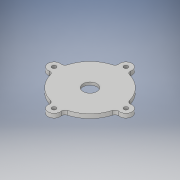
# Autodesk Inventor part: topPlateGB
Saved by Autodesk Inventor 2019 (Build 230136000, 136)
## iProperties
Created: 2019-10-26
Part Number: topPlateGB
Material: Generic
Document SubType Name: Modeling
Designer: test
Density: 1 g/cm^3
Appearance: Default
Author: test
Autodesk Inventor part; units mm, degrees
ref_plane "YZ Plane" through (0, 0, 0) normal (1, 0, 0) x (0, 1, 0)
ref_plane "XZ Plane" through (0, 0, 0) normal (0, 1, 0) x (-1, 0, 0)
ref_plane "XY Plane" through (0, 0, 0) normal (0, 0, 1) x (1, 0, 0)
sketch "Sketch1" plane through (0, 0, 0) normal (0, 1, 0) x (-1, 0, 0)
  circle A0 centre (33.02, 0) radius 1.778
  circle A1 centre (-33.02, 0) radius 1.778
  circle A2 centre (0, 33.02) radius 1.778
  circle A3 centre (0, -33.02) radius 1.778
  arc A4 (23.784909, -5.42928) -> (23.805274, -5.339279) centre (0, 0) ccw
  arc A5 (23.784909, -5.42928) -> (23.931742, -5.761352) centre (24.080982, -5.496864) ccw
  arc A6 (25.319623, -6.710384) -> (23.931742, -5.761352) centre (19.12448, -14.280927) ccw
  arc A7 (25.143294, -7.34352) -> (25.319623, -6.710384) centre (0, 0) ccw
  arc A8 (23.464649, -7.438525) -> (25.143294, -7.34352) centre (23.753261, 2.339492) ccw
  arc A9 (23.464649, -7.438525) -> (23.167304, -7.646894) centre (23.45569, -7.742082) ccw
  arc A10 (23.138215, -7.734466) -> (23.167304, -7.646894) centre (0, 0) ccw
  arc A11 (23.138215, -7.734466) -> (23.251792, -8.079331) centre (23.426239, -7.830744) ccw
  arc A12 (24.539969, -9.159828) -> (23.251792, -8.079331) centre (17.632615, -16.086687) ccw
  arc A13 (24.302432, -9.772633) -> (24.539969, -9.159828) centre (0, 0) ccw
  arc A14 (22.622558, -9.702644) -> (24.302432, -9.772633) centre (23.868193, 0) ccw
  arc A15 (22.622558, -9.702644) -> (22.306221, -9.880865) centre (22.583887, -10.003861) ccw
  arc A16 (22.268688, -9.965164) -> (22.306221, -9.880865) centre (0, 0) ccw
  arc A17 (22.268688, -9.965164) -> (22.347916, -10.319501) centre (22.545888, -10.08921) ccw
  arc A18 (23.523982, -11.521059) -> (22.347916, -10.319501) centre (15.970938, -17.737524) ccw
  arc A19 (23.227523, -12.10763) -> (23.523982, -11.521059) centre (0, 0) ccw
  arc A20 (21.562599, -11.873322) -> (23.227523, -12.10763) centre (23.753261, -2.339492) ccw
  arc A21 (21.562599, -11.873322) -> (21.230316, -12.019678) centre (21.49459, -12.169298) ccw
  arc A22 (21.184702, -12.099892) -> (21.230316, -12.019678) centre (0, 0) ccw
  arc A23 (21.184702, -12.099892) -> (21.228816, -12.460288) centre (21.448408, -12.250511) ccw
  arc A24 (22.281447, -13.771335) -> (21.228816, -12.460288) centre (14.155452, -19.217539) ccw
  arc A25 (21.928921, -14.326024) -> (22.281447, -13.771335) centre (0, 0) ccw
  arc A26 (20.29498, -13.929653) -> (21.928921, -14.326024) centre (23.409572, -4.656453) ccw
  arc A27 (20.29498, -13.929653) -> (19.949952, -14.042734) centre (20.198288, -14.217538) ccw
  arc A28 (19.896695, -14.118092) -> (19.949952, -14.042734) centre (0, 0) ccw
  arc A29 (19.896695, -14.118092) -> (19.905272, -14.481076) centre (20.144368, -14.293833) ccw
  arc A30 (20.824328, -15.888986) -> (19.905272, -14.481076) centre (12.203642, -20.512478) ccw
  arc A31 (20.419132, -16.40645) -> (20.824328, -15.888986) centre (0, 0) ccw
  arc A32 (18.831909, -15.851834) -> (20.419132, -16.40645) centre (22.840436, -6.928571) ccw
  arc A33 (18.831909, -15.851834) -> (18.477459, -15.930552) centre (18.707465, -16.128855) ccw
  arc A34 (18.417072, -16.000326) -> (18.477459, -15.930552) centre (0, 0) ccw
  arc A35 (18.417072, -16.000326) -> (18.390029, -16.362404) centre (18.646326, -16.199497) ccw
  arc A36 (19.166661, -17.853618) -> (18.390029, -16.362404) centre (10.134303, -21.609871) ccw
  arc A37 (18.712695, -18.328873) -> (19.166661, -17.853618) centre (0, 0) ccw
  arc A38 (17.187477, -17.621353) -> (18.712695, -18.328873) centre (22.051335, -9.133962) ccw
  arc A39 (17.187477, -17.621353) -> (16.827018, -17.66495) centre (17.036479, -17.884842) ccw
  arc A40 (16.760082, -17.728469) -> (16.827018, -17.66495) centre (0, 0) ccw
  arc A41 (16.760082, -17.728469) -> (16.69768, -18.086153) centre (16.968711, -17.949152) ccw
  arc A42 (17.324407, -19.646309) -> (16.69768, -18.086153) centre (7.967366, -22.499149) ccw
  arc A43 (16.826044, -20.07478) -> (17.324407, -19.646309) centre (0, 0) ccw
  arc A44 (15.37752, -19.221168) -> (16.826044, -20.07478) centre (21.049867, -11.251388) ccw
  arc A45 (15.37752, -19.221168) -> (15.014523, -19.229224) centre (15.201423, -19.468589) ccw
  arc A46 (14.941684, -19.285877) -> (15.014523, -19.229224) centre (0, 0) ccw
  arc A47 (14.941684, -19.285877) -> (14.844523, -19.635722) centre (15.127677, -19.525946) ccw
  arc A48 (15.315311, -21.249795) -> (14.844523, -19.635722) centre (5.723699, -23.171748) ccw
  arc A49 (14.77735, -21.627355) -> (15.315311, -21.249795) centre (0, 0) ccw
  arc A50 (13.419469, -20.635874) -> (14.77735, -21.627355) centre (19.845677, -13.260457) ccw
  arc A51 (13.419469, -20.635874) -> (13.05743, -20.608311) centre (13.219969, -20.864842) ccw
  arc A52 (12.979389, -20.657551) -> (13.05743, -20.608311) centre (0, 0) ccw
  arc A53 (12.979389, -20.657551) -> (12.848405, -20.996188) centre (13.140956, -20.914695) ccw
  arc A54 (13.158719, -22.648635) -> (12.848405, -20.996188) centre (3.424909, -23.62119) ccw
  arc A55 (12.586341, -22.971647) -> (13.158719, -22.648635) centre (0, 0) ccw
  arc A56 (11.332181, -21.851844) -> (12.586341, -22.971647) centre (18.450362, -15.141821) ccw
  arc A57 (11.332181, -21.851844) -> (10.974588, -21.788928) centre (11.111199, -22.060156) ccw
  arc A58 (10.892096, -21.830282) -> (10.974588, -21.788928) centre (0, 0) ccw
  arc A59 (10.892096, -21.830282) -> (10.728551, -22.15445) centre (11.02768, -22.102024) ccw
  arc A60 (10.875402, -23.829355) -> (10.728551, -22.15445) centre (1.093136, -23.843147) ccw
  arc A61 (10.274119, -24.094709) -> (10.875402, -23.829355) centre (0, 0) ccw
  arc A62 (9.135758, -22.85737) -> (10.274119, -24.094709) centre (16.877361, -16.877361) ccw
  arc A63 (9.135758, -22.85737) -> (8.786054, -22.759706) centre (8.895422, -23.043018) ccw
  arc A64 (8.699906, -22.792775) -> (8.786054, -22.759706) centre (0, 0) ccw
  arc A65 (8.699906, -22.792775) -> (8.505374, -23.099352) centre (8.808202, -23.076499) ccw
  arc A66 (8.487348, -24.780586) -> (8.505374, -23.099352) centre (-1.249165, -23.835482) ccw
  arc A67 (7.862952, -24.985726) -> (8.487348, -24.780586) centre (0, 0) ccw
  arc A68 (6.851353, -23.642766) -> (7.862952, -24.985726) centre (15.141821, -18.450362) ccw
  arc A69 (6.851353, -23.642766) -> (6.512905, -23.511296) centre (6.593977, -23.803963) ccw
  arc A70 (6.42393, -23.535762) -> (6.512905, -23.511296) centre (0, 0) ccw
  arc A71 (6.42393, -23.535762) -> (6.200286, -23.821794) centre (6.503895, -23.828734) ccw
  arc A72 (6.017557, -25.493167) -> (6.200286, -23.821794) centre (-3.579436, -23.598268) ccw
  arc A73 (5.37606, -25.636117) -> (6.017557, -25.493167) centre (0, 0) ccw
  arc A74 (4.500966, -24.20047) -> (5.37606, -25.636117) centre (13.260457, -19.845677) ccw
  arc A75 (4.500966, -24.20047) -> (4.177034, -24.036459) centre (4.229029, -24.335663) ccw
  arc A76 (4.086089, -24.052086) -> (4.177034, -24.036459) centre (0, 0) ccw
  arc A77 (4.086089, -24.052086) -> (3.835486, -24.31482) centre (4.136953, -24.351485) ccw
  arc A78 (3.489814, -25.960234) -> (3.835486, -24.31482) centre (-5.875234, -23.13379) ccw
  arc A79 (2.837394, -26.039619) -> (3.489814, -25.960234) centre (0, 0) ccw
  arc A80 (2.107231, -24.52511) -> (2.837394, -26.039619) centre (11.251388, -21.049867) ccw
  arc A81 (2.107231, -24.52511) -> (1.800935, -24.330138) centre (1.823353, -24.632998) ccw
  arc A82 (1.708897, -24.336775) -> (1.800935, -24.330138) centre (0, 0) ccw
  arc A83 (1.708897, -24.336775) -> (1.433747, -24.573681) centre (1.730169, -24.639718) ccw
  arc A84 (0.928462, -26.17729) -> (1.433747, -24.573681) centre (-8.114452, -22.446521) ccw
  arc A85 (0.271403, -26.192344) -> (0.928462, -26.17729) centre (0, 0) ccw
  arc A86 (-0.306797, -24.613559) -> (0.271403, -26.192344) centre (9.133962, -22.051335) ccw
  arc A87 (-0.306797, -24.613559) -> (-0.592507, -24.389504) centre (-0.599883, -24.693103) ccw
  arc A88 (-0.684753, -24.387088) -> (-0.592507, -24.389504) centre (0, 0) ccw
  arc A89 (-0.684753, -24.387088) -> (-0.981798, -24.595884) centre (-0.693277, -24.690658) ccw
  arc A90 (-1.641832, -26.142244) -> (-0.981798, -24.595884) centre (-10.275522, -21.543079) ccw
  arc A91 (-2.297203, -26.092823) -> (-1.641832, -26.142244) centre (0, 0) ccw
  arc A92 (-2.71787, -24.464967) -> (-2.297203, -26.092823) centre (6.928571, -22.840436) ccw
  arc A93 (-2.71787, -24.464967) -> (-2.980244, -24.213986) centre (-3.017342, -24.5154) ccw
  arc A94 (-3.071808, -24.20254) -> (-2.980244, -24.213986) centre (0, 0) ccw
  arc A95 (-3.071808, -24.20254) -> (-3.387889, -24.381215) centre (-3.110046, -24.503812) ccw
  arc A96 (-4.196314, -25.855434) -> (-3.387889, -24.381215) centre (-12.337634, -20.432166) ccw
  arc A97 (-4.843685, -25.742013) -> (-4.196314, -25.855434) centre (0, 0) ccw
  arc A98 (-5.102769, -24.080764) -> (-4.843685, -25.742013) centre (4.656453, -23.409572) ccw
  arc A99 (-5.102769, -24.080764) -> (-5.339279, -23.805274) centre (-5.405742, -24.101601) ccw
  arc A100 (-5.42928, -23.784909) -> (-5.339279, -23.805274) centre (0, 0) ccw
  arc A101 (-5.42928, -23.784909) -> (-5.761352, -23.931742) centre (-5.496864, -24.080982) ccw
  arc A102 (-6.710384, -25.319623) -> (-5.761352, -23.931742) centre (-14.280927, -19.12448) ccw
  arc A103 (-7.34352, -25.143294) -> (-6.710384, -25.319623) centre (0, 0) ccw
  arc A104 (-7.438525, -23.464649) -> (-7.34352, -25.143294) centre (2.339492, -23.753261) ccw
  arc A105 (-7.438525, -23.464649) -> (-7.646894, -23.167304) centre (-7.742082, -23.45569) ccw
  arc A106 (-7.734466, -23.138215) -> (-7.646894, -23.167304) centre (0, 0) ccw
  arc A107 (-7.734466, -23.138215) -> (-8.079331, -23.251792) centre (-7.830744, -23.426239) ccw
  arc A108 (-9.159828, -24.539969) -> (-8.079331, -23.251792) centre (-16.086687, -17.632615) ccw
  arc A109 (-9.772633, -24.302432) -> (-9.159828, -24.539969) centre (0, 0) ccw
  arc A110 (-9.702644, -22.622558) -> (-9.772633, -24.302432) centre (0, -23.868193) ccw
  arc A111 (-9.702644, -22.622558) -> (-9.880865, -22.306221) centre (-10.003861, -22.583887) ccw
  arc A112 (-9.965164, -22.268688) -> (-9.880865, -22.306221) centre (0, 0) ccw
  arc A113 (-9.965164, -22.268688) -> (-10.319501, -22.347916) centre (-10.08921, -22.545888) ccw
  arc A114 (-11.521059, -23.523982) -> (-10.319501, -22.347916) centre (-17.737524, -15.970938) ccw
  arc A115 (-12.10763, -23.227523) -> (-11.521059, -23.523982) centre (0, 0) ccw
  arc A116 (-11.873322, -21.562599) -> (-12.10763, -23.227523) centre (-2.339492, -23.753261) ccw
  arc A117 (-11.873322, -21.562599) -> (-12.019678, -21.230316) centre (-12.169298, -21.49459) ccw
  arc A118 (-12.099892, -21.184702) -> (-12.019678, -21.230316) centre (0, 0) ccw
  arc A119 (-12.099892, -21.184702) -> (-12.460288, -21.228816) centre (-12.250511, -21.448408) ccw
  arc A120 (-13.771335, -22.281447) -> (-12.460288, -21.228816) centre (-19.217539, -14.155452) ccw
  arc A121 (-14.326024, -21.928921) -> (-13.771335, -22.281447) centre (0, 0) ccw
  arc A122 (-13.929653, -20.29498) -> (-14.326024, -21.928921) centre (-4.656453, -23.409572) ccw
  arc A123 (-13.929653, -20.29498) -> (-14.042734, -19.949952) centre (-14.217538, -20.198288) ccw
  arc A124 (-14.118092, -19.896695) -> (-14.042734, -19.949952) centre (0, 0) ccw
  arc A125 (-14.118092, -19.896695) -> (-14.481076, -19.905272) centre (-14.293833, -20.144368) ccw
  arc A126 (-15.888986, -20.824328) -> (-14.481076, -19.905272) centre (-20.512478, -12.203642) ccw
  arc A127 (-16.40645, -20.419132) -> (-15.888986, -20.824328) centre (0, 0) ccw
  arc A128 (-15.851834, -18.831909) -> (-16.40645, -20.419132) centre (-6.928571, -22.840436) ccw
  arc A129 (-15.851834, -18.831909) -> (-15.930552, -18.477459) centre (-16.128855, -18.707465) ccw
  arc A130 (-16.000326, -18.417072) -> (-15.930552, -18.477459) centre (0, 0) ccw
  arc A131 (-16.000326, -18.417072) -> (-16.362404, -18.390029) centre (-16.199497, -18.646326) ccw
  arc A132 (-17.853618, -19.166661) -> (-16.362404, -18.390029) centre (-21.609871, -10.134303) ccw
  arc A133 (-18.328873, -18.712695) -> (-17.853618, -19.166661) centre (0, 0) ccw
  arc A134 (-17.621353, -17.187477) -> (-18.328873, -18.712695) centre (-9.133962, -22.051335) ccw
  arc A135 (-17.621353, -17.187477) -> (-17.66495, -16.827018) centre (-17.884842, -17.036479) ccw
  arc A136 (-17.728469, -16.760082) -> (-17.66495, -16.827018) centre (0, 0) ccw
  arc A137 (-17.728469, -16.760082) -> (-18.086153, -16.69768) centre (-17.949152, -16.968711) ccw
  arc A138 (-19.646309, -17.324407) -> (-18.086153, -16.69768) centre (-22.499149, -7.967366) ccw
  arc A139 (-20.07478, -16.826044) -> (-19.646309, -17.324407) centre (0, 0) ccw
  arc A140 (-19.221168, -15.37752) -> (-20.07478, -16.826044) centre (-11.251388, -21.049867) ccw
  arc A141 (-19.221168, -15.37752) -> (-19.229224, -15.014523) centre (-19.468589, -15.201423) ccw
  arc A142 (-19.285877, -14.941684) -> (-19.229224, -15.014523) centre (0, 0) ccw
  arc A143 (-19.285877, -14.941684) -> (-19.635722, -14.844523) centre (-19.525946, -15.127677) ccw
  arc A144 (-21.249795, -15.315311) -> (-19.635722, -14.844523) centre (-23.171748, -5.723699) ccw
  arc A145 (-21.627355, -14.77735) -> (-21.249795, -15.315311) centre (0, 0) ccw
  arc A146 (-20.635874, -13.419469) -> (-21.627355, -14.77735) centre (-13.260457, -19.845677) ccw
  arc A147 (-20.635874, -13.419469) -> (-20.608311, -13.05743) centre (-20.864842, -13.219969) ccw
  arc A148 (-20.657551, -12.979389) -> (-20.608311, -13.05743) centre (0, 0) ccw
  arc A149 (-20.657551, -12.979389) -> (-20.996188, -12.848405) centre (-20.914695, -13.140956) ccw
  arc A150 (-22.648635, -13.158719) -> (-20.996188, -12.848405) centre (-23.62119, -3.424909) ccw
  arc A151 (-22.971647, -12.586341) -> (-22.648635, -13.158719) centre (0, 0) ccw
  arc A152 (-21.851844, -11.332181) -> (-22.971647, -12.586341) centre (-15.141821, -18.450362) ccw
  arc A153 (-21.851844, -11.332181) -> (-21.788928, -10.974588) centre (-22.060156, -11.111199) ccw
  arc A154 (-21.830282, -10.892096) -> (-21.788928, -10.974588) centre (0, 0) ccw
  arc A155 (-21.830282, -10.892096) -> (-22.15445, -10.728551) centre (-22.102024, -11.02768) ccw
  arc A156 (-23.829355, -10.875402) -> (-22.15445, -10.728551) centre (-23.843147, -1.093136) ccw
  arc A157 (-24.094709, -10.274119) -> (-23.829355, -10.875402) centre (0, 0) ccw
  arc A158 (-22.85737, -9.135758) -> (-24.094709, -10.274119) centre (-16.877361, -16.877361) ccw
  arc A159 (-22.85737, -9.135758) -> (-22.759706, -8.786054) centre (-23.043018, -8.895422) ccw
  arc A160 (-22.792775, -8.699906) -> (-22.759706, -8.786054) centre (0, 0) ccw
  arc A161 (-22.792775, -8.699906) -> (-23.099352, -8.505374) centre (-23.076499, -8.808202) ccw
  arc A162 (-24.780586, -8.487348) -> (-23.099352, -8.505374) centre (-23.835482, 1.249165) ccw
  arc A163 (-24.985726, -7.862952) -> (-24.780586, -8.487348) centre (0, 0) ccw
  arc A164 (-23.642766, -6.851353) -> (-24.985726, -7.862952) centre (-18.450362, -15.141821) ccw
  arc A165 (-23.642766, -6.851353) -> (-23.511296, -6.512905) centre (-23.803963, -6.593977) ccw
  arc A166 (-23.535762, -6.42393) -> (-23.511296, -6.512905) centre (0, 0) ccw
  arc A167 (-23.535762, -6.42393) -> (-23.821794, -6.200286) centre (-23.828734, -6.503895) ccw
  arc A168 (-25.493167, -6.017557) -> (-23.821794, -6.200286) centre (-23.598268, 3.579436) ccw
  arc A169 (-25.636117, -5.37606) -> (-25.493167, -6.017557) centre (0, 0) ccw
  arc A170 (-24.20047, -4.500966) -> (-25.636117, -5.37606) centre (-19.845677, -13.260457) ccw
  arc A171 (-24.20047, -4.500966) -> (-24.036459, -4.177034) centre (-24.335663, -4.229029) ccw
  arc A172 (-24.052086, -4.086089) -> (-24.036459, -4.177034) centre (0, 0) ccw
  arc A173 (-24.052086, -4.086089) -> (-24.31482, -3.835486) centre (-24.351485, -4.136953) ccw
  arc A174 (-25.960234, -3.489814) -> (-24.31482, -3.835486) centre (-23.13379, 5.875234) ccw
  arc A175 (-26.039619, -2.837394) -> (-25.960234, -3.489814) centre (0, 0) ccw
  arc A176 (-24.52511, -2.107231) -> (-26.039619, -2.837394) centre (-21.049867, -11.251388) ccw
  arc A177 (-24.52511, -2.107231) -> (-24.330138, -1.800935) centre (-24.632998, -1.823353) ccw
  arc A178 (-24.336775, -1.708897) -> (-24.330138, -1.800935) centre (0, 0) ccw
  arc A179 (-24.336775, -1.708897) -> (-24.573681, -1.433747) centre (-24.639718, -1.730169) ccw
  arc A180 (-26.17729, -0.928462) -> (-24.573681, -1.433747) centre (-22.446521, 8.114452) ccw
  arc A181 (-26.192344, -0.271403) -> (-26.17729, -0.928462) centre (0, 0) ccw
  arc A182 (-24.613559, 0.306797) -> (-26.192344, -0.271403) centre (-22.051335, -9.133962) ccw
  arc A183 (-24.613559, 0.306797) -> (-24.389504, 0.592507) centre (-24.693103, 0.599883) ccw
  arc A184 (-24.387088, 0.684753) -> (-24.389504, 0.592507) centre (0, 0) ccw
  arc A185 (-24.387088, 0.684753) -> (-24.595884, 0.981798) centre (-24.690658, 0.693277) ccw
  arc A186 (-26.142244, 1.641832) -> (-24.595884, 0.981798) centre (-21.543079, 10.275522) ccw
  arc A187 (-26.092823, 2.297203) -> (-26.142244, 1.641832) centre (0, 0) ccw
  arc A188 (-24.464967, 2.71787) -> (-26.092823, 2.297203) centre (-22.840436, -6.928571) ccw
  arc A189 (-24.464967, 2.71787) -> (-24.213986, 2.980244) centre (-24.5154, 3.017342) ccw
  arc A190 (-24.20254, 3.071808) -> (-24.213986, 2.980244) centre (0, 0) ccw
  arc A191 (-24.20254, 3.071808) -> (-24.381215, 3.387889) centre (-24.503812, 3.110046) ccw
  arc A192 (-25.855434, 4.196314) -> (-24.381215, 3.387889) centre (-20.432166, 12.337634) ccw
  arc A193 (-25.742013, 4.843685) -> (-25.855434, 4.196314) centre (0, 0) ccw
  arc A194 (-24.080764, 5.102769) -> (-25.742013, 4.843685) centre (-23.409572, -4.656453) ccw
  arc A195 (-24.080764, 5.102769) -> (-23.805274, 5.339279) centre (-24.101601, 5.405742) ccw
  arc A196 (-23.784909, 5.42928) -> (-23.805274, 5.339279) centre (0, 0) ccw
  arc A197 (-23.784909, 5.42928) -> (-23.931742, 5.761352) centre (-24.080982, 5.496864) ccw
  arc A198 (-25.319623, 6.710384) -> (-23.931742, 5.761352) centre (-19.12448, 14.280927) ccw
  arc A199 (-25.143294, 7.34352) -> (-25.319623, 6.710384) centre (0, 0) ccw
  arc A200 (-23.464649, 7.438525) -> (-25.143294, 7.34352) centre (-23.753261, -2.339492) ccw
  arc A201 (-23.464649, 7.438525) -> (-23.167304, 7.646894) centre (-23.45569, 7.742082) ccw
  arc A202 (-23.138215, 7.734466) -> (-23.167304, 7.646894) centre (0, 0) ccw
  arc A203 (-23.138215, 7.734466) -> (-23.251792, 8.079331) centre (-23.426239, 7.830744) ccw
  arc A204 (-24.539969, 9.159828) -> (-23.251792, 8.079331) centre (-17.632615, 16.086687) ccw
  arc A205 (-24.302432, 9.772633) -> (-24.539969, 9.159828) centre (0, 0) ccw
  arc A206 (-22.622558, 9.702644) -> (-24.302432, 9.772633) centre (-23.868193, 0) ccw
  arc A207 (-22.622558, 9.702644) -> (-22.306221, 9.880865) centre (-22.583887, 10.003861) ccw
  arc A208 (-22.268688, 9.965164) -> (-22.306221, 9.880865) centre (0, 0) ccw
  arc A209 (-22.268688, 9.965164) -> (-22.347916, 10.319501) centre (-22.545888, 10.08921) ccw
  arc A210 (-23.523982, 11.521059) -> (-22.347916, 10.319501) centre (-15.970938, 17.737524) ccw
  arc A211 (-23.227523, 12.10763) -> (-23.523982, 11.521059) centre (0, 0) ccw
  arc A212 (-21.562599, 11.873322) -> (-23.227523, 12.10763) centre (-23.753261, 2.339492) ccw
  arc A213 (-21.562599, 11.873322) -> (-21.230316, 12.019678) centre (-21.49459, 12.169298) ccw
  arc A214 (-21.184702, 12.099892) -> (-21.230316, 12.019678) centre (0, 0) ccw
  arc A215 (-21.184702, 12.099892) -> (-21.228816, 12.460288) centre (-21.448408, 12.250511) ccw
  arc A216 (-22.281447, 13.771335) -> (-21.228816, 12.460288) centre (-14.155452, 19.217539) ccw
  arc A217 (-21.928921, 14.326024) -> (-22.281447, 13.771335) centre (0, 0) ccw
  arc A218 (-20.29498, 13.929653) -> (-21.928921, 14.326024) centre (-23.409572, 4.656453) ccw
  arc A219 (-20.29498, 13.929653) -> (-19.949952, 14.042734) centre (-20.198288, 14.217538) ccw
  arc A220 (-19.896695, 14.118092) -> (-19.949952, 14.042734) centre (0, 0) ccw
  arc A221 (-19.896695, 14.118092) -> (-19.905272, 14.481076) centre (-20.144368, 14.293833) ccw
  arc A222 (-20.824328, 15.888986) -> (-19.905272, 14.481076) centre (-12.203642, 20.512478) ccw
  arc A223 (-20.419132, 16.40645) -> (-20.824328, 15.888986) centre (0, 0) ccw
  arc A224 (-18.831909, 15.851834) -> (-20.419132, 16.40645) centre (-22.840436, 6.928571) ccw
  arc A225 (-18.831909, 15.851834) -> (-18.477459, 15.930552) centre (-18.707465, 16.128855) ccw
  arc A226 (-18.417072, 16.000326) -> (-18.477459, 15.930552) centre (0, 0) ccw
  arc A227 (-18.417072, 16.000326) -> (-18.390029, 16.362404) centre (-18.646326, 16.199497) ccw
  arc A228 (-19.166661, 17.853618) -> (-18.390029, 16.362404) centre (-10.134303, 21.609871) ccw
  arc A229 (-18.712695, 18.328873) -> (-19.166661, 17.853618) centre (0, 0) ccw
  arc A230 (-17.187477, 17.621353) -> (-18.712695, 18.328873) centre (-22.051335, 9.133962) ccw
  arc A231 (-17.187477, 17.621353) -> (-16.827018, 17.66495) centre (-17.036479, 17.884842) ccw
  arc A232 (-16.760082, 17.728469) -> (-16.827018, 17.66495) centre (0, 0) ccw
  arc A233 (-16.760082, 17.728469) -> (-16.69768, 18.086153) centre (-16.968711, 17.949152) ccw
  arc A234 (-17.324407, 19.646309) -> (-16.69768, 18.086153) centre (-7.967366, 22.499149) ccw
  arc A235 (-16.826044, 20.07478) -> (-17.324407, 19.646309) centre (0, 0) ccw
  arc A236 (-15.37752, 19.221168) -> (-16.826044, 20.07478) centre (-21.049867, 11.251388) ccw
  arc A237 (-15.37752, 19.221168) -> (-15.014523, 19.229224) centre (-15.201423, 19.468589) ccw
  arc A238 (-14.941684, 19.285877) -> (-15.014523, 19.229224) centre (0, 0) ccw
  arc A239 (-14.941684, 19.285877) -> (-14.844523, 19.635722) centre (-15.127677, 19.525946) ccw
  arc A240 (-15.315311, 21.249795) -> (-14.844523, 19.635722) centre (-5.723699, 23.171748) ccw
  arc A241 (-14.77735, 21.627355) -> (-15.315311, 21.249795) centre (0, 0) ccw
  arc A242 (-13.419469, 20.635874) -> (-14.77735, 21.627355) centre (-19.845677, 13.260457) ccw
  arc A243 (-13.419469, 20.635874) -> (-13.05743, 20.608311) centre (-13.219969, 20.864842) ccw
  arc A244 (-12.979389, 20.657551) -> (-13.05743, 20.608311) centre (0, 0) ccw
  arc A245 (-12.979389, 20.657551) -> (-12.848405, 20.996188) centre (-13.140956, 20.914695) ccw
  arc A246 (-13.158719, 22.648635) -> (-12.848405, 20.996188) centre (-3.424909, 23.62119) ccw
  arc A247 (-12.586341, 22.971647) -> (-13.158719, 22.648635) centre (0, 0) ccw
  arc A248 (-11.332181, 21.851844) -> (-12.586341, 22.971647) centre (-18.450362, 15.141821) ccw
  arc A249 (-11.332181, 21.851844) -> (-10.974588, 21.788928) centre (-11.111199, 22.060156) ccw
  arc A250 (-10.892096, 21.830282) -> (-10.974588, 21.788928) centre (0, 0) ccw
  arc A251 (-10.892096, 21.830282) -> (-10.728551, 22.15445) centre (-11.02768, 22.102024) ccw
  arc A252 (-10.875402, 23.829355) -> (-10.728551, 22.15445) centre (-1.093136, 23.843147) ccw
  arc A253 (-10.274119, 24.094709) -> (-10.875402, 23.829355) centre (0, 0) ccw
  arc A254 (-9.135758, 22.85737) -> (-10.274119, 24.094709) centre (-16.877361, 16.877361) ccw
  arc A255 (-9.135758, 22.85737) -> (-8.786054, 22.759706) centre (-8.895422, 23.043018) ccw
  arc A256 (-8.699906, 22.792775) -> (-8.786054, 22.759706) centre (0, 0) ccw
  arc A257 (-8.699906, 22.792775) -> (-8.505374, 23.099352) centre (-8.808202, 23.076499) ccw
  arc A258 (-8.487348, 24.780586) -> (-8.505374, 23.099352) centre (1.249165, 23.835482) ccw
  arc A259 (-7.862952, 24.985726) -> (-8.487348, 24.780586) centre (0, 0) ccw
  arc A260 (-6.851353, 23.642766) -> (-7.862952, 24.985726) centre (-15.141821, 18.450362) ccw
  arc A261 (-6.851353, 23.642766) -> (-6.512905, 23.511296) centre (-6.593977, 23.803963) ccw
  arc A262 (-6.42393, 23.535762) -> (-6.512905, 23.511296) centre (0, 0) ccw
  arc A263 (-6.42393, 23.535762) -> (-6.200286, 23.821794) centre (-6.503895, 23.828734) ccw
  arc A264 (-6.017557, 25.493167) -> (-6.200286, 23.821794) centre (3.579436, 23.598268) ccw
  arc A265 (-5.37606, 25.636117) -> (-6.017557, 25.493167) centre (0, 0) ccw
  arc A266 (-4.500966, 24.20047) -> (-5.37606, 25.636117) centre (-13.260457, 19.845677) ccw
  arc A267 (-4.500966, 24.20047) -> (-4.177034, 24.036459) centre (-4.229029, 24.335663) ccw
  arc A268 (-4.086089, 24.052086) -> (-4.177034, 24.036459) centre (0, 0) ccw
  arc A269 (-4.086089, 24.052086) -> (-3.835486, 24.31482) centre (-4.136953, 24.351485) ccw
  arc A270 (-3.489814, 25.960234) -> (-3.835486, 24.31482) centre (5.875234, 23.13379) ccw
  arc A271 (-2.837394, 26.039619) -> (-3.489814, 25.960234) centre (0, 0) ccw
  arc A272 (-2.107231, 24.52511) -> (-2.837394, 26.039619) centre (-11.251388, 21.049867) ccw
  arc A273 (-2.107231, 24.52511) -> (-1.800935, 24.330138) centre (-1.823353, 24.632998) ccw
  arc A274 (-1.708897, 24.336775) -> (-1.800935, 24.330138) centre (0, 0) ccw
  arc A275 (-1.708897, 24.336775) -> (-1.433747, 24.573681) centre (-1.730169, 24.639718) ccw
  arc A276 (-0.928462, 26.17729) -> (-1.433747, 24.573681) centre (8.114452, 22.446521) ccw
  arc A277 (-0.271403, 26.192344) -> (-0.928462, 26.17729) centre (0, 0) ccw
  arc A278 (0.306797, 24.613559) -> (-0.271403, 26.192344) centre (-9.133962, 22.051335) ccw
  arc A279 (0.306797, 24.613559) -> (0.592507, 24.389504) centre (0.599883, 24.693103) ccw
  arc A280 (0.684753, 24.387088) -> (0.592507, 24.389504) centre (0, 0) ccw
  arc A281 (0.684753, 24.387088) -> (0.981798, 24.595884) centre (0.693277, 24.690658) ccw
  arc A282 (1.641832, 26.142244) -> (0.981798, 24.595884) centre (10.275522, 21.543079) ccw
  arc A283 (2.297203, 26.092823) -> (1.641832, 26.142244) centre (0, 0) ccw
  arc A284 (2.71787, 24.464967) -> (2.297203, 26.092823) centre (-6.928571, 22.840436) ccw
  arc A285 (2.71787, 24.464967) -> (2.980244, 24.213986) centre (3.017342, 24.5154) ccw
  arc A286 (3.071808, 24.20254) -> (2.980244, 24.213986) centre (0, 0) ccw
  arc A287 (3.071808, 24.20254) -> (3.387889, 24.381215) centre (3.110046, 24.503812) ccw
  arc A288 (4.196314, 25.855434) -> (3.387889, 24.381215) centre (12.337634, 20.432166) ccw
  arc A289 (4.843685, 25.742013) -> (4.196314, 25.855434) centre (0, 0) ccw
  arc A290 (5.102769, 24.080764) -> (4.843685, 25.742013) centre (-4.656453, 23.409572) ccw
  arc A291 (5.102769, 24.080764) -> (5.339279, 23.805274) centre (5.405742, 24.101601) ccw
  arc A292 (5.42928, 23.784909) -> (5.339279, 23.805274) centre (0, 0) ccw
  arc A293 (5.42928, 23.784909) -> (5.761352, 23.931742) centre (5.496864, 24.080982) ccw
  arc A294 (6.710384, 25.319623) -> (5.761352, 23.931742) centre (14.280927, 19.12448) ccw
  arc A295 (7.34352, 25.143294) -> (6.710384, 25.319623) centre (0, 0) ccw
  arc A296 (7.438525, 23.464649) -> (7.34352, 25.143294) centre (-2.339492, 23.753261) ccw
  arc A297 (7.438525, 23.464649) -> (7.646894, 23.167304) centre (7.742082, 23.45569) ccw
  arc A298 (7.734466, 23.138215) -> (7.646894, 23.167304) centre (0, 0) ccw
  arc A299 (7.734466, 23.138215) -> (8.079331, 23.251792) centre (7.830744, 23.426239) ccw
  arc A300 (9.159828, 24.539969) -> (8.079331, 23.251792) centre (16.086687, 17.632615) ccw
  arc A301 (9.772633, 24.302432) -> (9.159828, 24.539969) centre (0, 0) ccw
  arc A302 (9.702644, 22.622558) -> (9.772633, 24.302432) centre (0, 23.868193) ccw
  arc A303 (9.702644, 22.622558) -> (9.880865, 22.306221) centre (10.003861, 22.583887) ccw
  arc A304 (9.965164, 22.268688) -> (9.880865, 22.306221) centre (0, 0) ccw
  arc A305 (9.965164, 22.268688) -> (10.319501, 22.347916) centre (10.08921, 22.545888) ccw
  arc A306 (11.521059, 23.523982) -> (10.319501, 22.347916) centre (17.737524, 15.970938) ccw
  arc A307 (12.10763, 23.227523) -> (11.521059, 23.523982) centre (0, 0) ccw
  arc A308 (11.873322, 21.562599) -> (12.10763, 23.227523) centre (2.339492, 23.753261) ccw
  arc A309 (11.873322, 21.562599) -> (12.019678, 21.230316) centre (12.169298, 21.49459) ccw
  arc A310 (12.099892, 21.184702) -> (12.019678, 21.230316) centre (0, 0) ccw
  arc A311 (12.099892, 21.184702) -> (12.460288, 21.228816) centre (12.250511, 21.448408) ccw
  arc A312 (13.771335, 22.281447) -> (12.460288, 21.228816) centre (19.217539, 14.155452) ccw
  arc A313 (14.326024, 21.928921) -> (13.771335, 22.281447) centre (0, 0) ccw
  arc A314 (13.929653, 20.29498) -> (14.326024, 21.928921) centre (4.656453, 23.409572) ccw
  arc A315 (13.929653, 20.29498) -> (14.042734, 19.949952) centre (14.217538, 20.198288) ccw
  arc A316 (14.118092, 19.896695) -> (14.042734, 19.949952) centre (0, 0) ccw
  arc A317 (14.118092, 19.896695) -> (14.481076, 19.905272) centre (14.293833, 20.144368) ccw
  arc A318 (15.888986, 20.824328) -> (14.481076, 19.905272) centre (20.512478, 12.203642) ccw
  arc A319 (16.40645, 20.419132) -> (15.888986, 20.824328) centre (0, 0) ccw
  arc A320 (15.851834, 18.831909) -> (16.40645, 20.419132) centre (6.928571, 22.840436) ccw
  arc A321 (15.851834, 18.831909) -> (15.930552, 18.477459) centre (16.128855, 18.707465) ccw
  arc A322 (16.000326, 18.417072) -> (15.930552, 18.477459) centre (0, 0) ccw
  arc A323 (16.000326, 18.417072) -> (16.362404, 18.390029) centre (16.199497, 18.646326) ccw
  arc A324 (17.853618, 19.166661) -> (16.362404, 18.390029) centre (21.609871, 10.134303) ccw
  arc A325 (18.328873, 18.712695) -> (17.853618, 19.166661) centre (0, 0) ccw
  arc A326 (17.621353, 17.187477) -> (18.328873, 18.712695) centre (9.133962, 22.051335) ccw
  arc A327 (17.621353, 17.187477) -> (17.66495, 16.827018) centre (17.884842, 17.036479) ccw
  arc A328 (17.728469, 16.760082) -> (17.66495, 16.827018) centre (0, 0) ccw
  arc A329 (17.728469, 16.760082) -> (18.086153, 16.69768) centre (17.949152, 16.968711) ccw
  arc A330 (19.646309, 17.324407) -> (18.086153, 16.69768) centre (22.499149, 7.967366) ccw
  arc A331 (20.07478, 16.826044) -> (19.646309, 17.324407) centre (0, 0) ccw
  arc A332 (19.221168, 15.37752) -> (20.07478, 16.826044) centre (11.251388, 21.049867) ccw
  arc A333 (19.221168, 15.37752) -> (19.229224, 15.014523) centre (19.468589, 15.201423) ccw
  arc A334 (19.285877, 14.941684) -> (19.229224, 15.014523) centre (0, 0) ccw
  arc A335 (19.285877, 14.941684) -> (19.635722, 14.844523) centre (19.525946, 15.127677) ccw
  arc A336 (21.249795, 15.315311) -> (19.635722, 14.844523) centre (23.171748, 5.723699) ccw
  arc A337 (21.627355, 14.77735) -> (21.249795, 15.315311) centre (0, 0) ccw
  arc A338 (20.635874, 13.419469) -> (21.627355, 14.77735) centre (13.260457, 19.845677) ccw
  arc A339 (20.635874, 13.419469) -> (20.608311, 13.05743) centre (20.864842, 13.219969) ccw
  arc A340 (20.657551, 12.979389) -> (20.608311, 13.05743) centre (0, 0) ccw
  arc A341 (20.657551, 12.979389) -> (20.996188, 12.848405) centre (20.914695, 13.140956) ccw
  arc A342 (22.648635, 13.158719) -> (20.996188, 12.848405) centre (23.62119, 3.424909) ccw
  arc A343 (22.971647, 12.586341) -> (22.648635, 13.158719) centre (0, 0) ccw
  arc A344 (21.851844, 11.332181) -> (22.971647, 12.586341) centre (15.141821, 18.450362) ccw
  arc A345 (21.851844, 11.332181) -> (21.788928, 10.974588) centre (22.060156, 11.111199) ccw
  arc A346 (21.830282, 10.892096) -> (21.788928, 10.974588) centre (0, 0) ccw
  arc A347 (21.830282, 10.892096) -> (22.15445, 10.728551) centre (22.102024, 11.02768) ccw
  arc A348 (23.829355, 10.875402) -> (22.15445, 10.728551) centre (23.843147, 1.093136) ccw
  arc A349 (24.094709, 10.274119) -> (23.829355, 10.875402) centre (0, 0) ccw
  arc A350 (22.85737, 9.135758) -> (24.094709, 10.274119) centre (16.877361, 16.877361) ccw
  arc A351 (22.85737, 9.135758) -> (22.759706, 8.786054) centre (23.043018, 8.895422) ccw
  arc A352 (22.792775, 8.699906) -> (22.759706, 8.786054) centre (0, 0) ccw
  arc A353 (22.792775, 8.699906) -> (23.099352, 8.505374) centre (23.076499, 8.808202) ccw
  arc A354 (24.780586, 8.487348) -> (23.099352, 8.505374) centre (23.835482, -1.249165) ccw
  arc A355 (24.985726, 7.862952) -> (24.780586, 8.487348) centre (0, 0) ccw
  arc A356 (23.642766, 6.851353) -> (24.985726, 7.862952) centre (18.450362, 15.141821) ccw
  arc A357 (23.642766, 6.851353) -> (23.511296, 6.512905) centre (23.803963, 6.593977) ccw
  arc A358 (23.535762, 6.42393) -> (23.511296, 6.512905) centre (0, 0) ccw
  arc A359 (23.535762, 6.42393) -> (23.821794, 6.200286) centre (23.828734, 6.503895) ccw
  arc A360 (25.493167, 6.017557) -> (23.821794, 6.200286) centre (23.598268, -3.579436) ccw
  arc A361 (25.636117, 5.37606) -> (25.493167, 6.017557) centre (0, 0) ccw
  arc A362 (24.20047, 4.500966) -> (25.636117, 5.37606) centre (19.845677, 13.260457) ccw
  arc A363 (24.20047, 4.500966) -> (24.036459, 4.177034) centre (24.335663, 4.229029) ccw
  arc A364 (24.052086, 4.086089) -> (24.036459, 4.177034) centre (0, 0) ccw
  arc A365 (24.052086, 4.086089) -> (24.31482, 3.835486) centre (24.351485, 4.136953) ccw
  arc A366 (25.960234, 3.489814) -> (24.31482, 3.835486) centre (23.13379, -5.875234) ccw
  arc A367 (26.039619, 2.837394) -> (25.960234, 3.489814) centre (0, 0) ccw
  arc A368 (24.52511, 2.107231) -> (26.039619, 2.837394) centre (21.049867, 11.251388) ccw
  arc A369 (24.52511, 2.107231) -> (24.330138, 1.800935) centre (24.632998, 1.823353) ccw
  arc A370 (24.336775, 1.708897) -> (24.330138, 1.800935) centre (0, 0) ccw
  arc A371 (24.336775, 1.708897) -> (24.573681, 1.433747) centre (24.639718, 1.730169) ccw
  arc A372 (26.17729, 0.928462) -> (24.573681, 1.433747) centre (22.446521, -8.114452) ccw
  arc A373 (26.192344, 0.271403) -> (26.17729, 0.928462) centre (0, 0) ccw
  arc A374 (24.613559, -0.306797) -> (26.192344, 0.271403) centre (22.051335, 9.133962) ccw
  arc A375 (24.613559, -0.306797) -> (24.389504, -0.592507) centre (24.693103, -0.599883) ccw
  arc A376 (24.387088, -0.684753) -> (24.389504, -0.592507) centre (0, 0) ccw
  arc A377 (24.387088, -0.684753) -> (24.595884, -0.981798) centre (24.690658, -0.693277) ccw
  arc A378 (26.142244, -1.641832) -> (24.595884, -0.981798) centre (21.543079, -10.275522) ccw
  arc A379 (26.092823, -2.297203) -> (26.142244, -1.641832) centre (0, 0) ccw
  arc A380 (24.464967, -2.71787) -> (26.092823, -2.297203) centre (22.840436, 6.928571) ccw
  arc A381 (24.464967, -2.71787) -> (24.213986, -2.980244) centre (24.5154, -3.017342) ccw
  arc A382 (24.20254, -3.071808) -> (24.213986, -2.980244) centre (0, 0) ccw
  arc A383 (24.20254, -3.071808) -> (24.381215, -3.387889) centre (24.503812, -3.110046) ccw
  arc A384 (25.855434, -4.196314) -> (24.381215, -3.387889) centre (20.432166, -12.337634) ccw
  arc A385 (25.742013, -4.843685) -> (25.855434, -4.196314) centre (0, 0) ccw
  arc A386 (24.080764, -5.102769) -> (25.742013, -4.843685) centre (23.409572, 4.656453) ccw
  arc A387 (24.080764, -5.102769) -> (23.805274, -5.339279) centre (24.101601, -5.405742) ccw
  arc A388 (29.192502, 4.071364) -> (4.071364, 29.192502) centre (0, 0) ccw
  arc A389 (4.071364, 29.192502) -> (-4.071364, 29.192502) centre (0, 33.02) ccw
  arc A390 (-4.071364, 29.192502) -> (-29.192502, 4.071364) centre (0, 0) ccw
  arc A391 (-29.192502, 4.071364) -> (-29.192502, -4.071364) centre (-33.02, 0) ccw
  arc A392 (-29.192502, -4.071364) -> (-4.071364, -29.192502) centre (0, 0) ccw
  arc A393 (-4.071364, -29.192502) -> (4.071364, -29.192502) centre (0, -33.02) ccw
  arc A394 (4.071364, -29.192502) -> (29.192502, -4.071364) centre (0, 0) ccw
  arc A395 (29.192502, -4.071364) -> (29.192502, 4.071364) centre (33.02, 0) ccw
  point P0 (0, 0)
  constraints: 784 point on circle, 396 centre point
extrude "Extrusion1" add sketch "Sketch1" along normal blind 3.81
sketch "Sketch2" plane through (0, 3.81, 0) normal (0, 1, 0) x (1, 0, 0)
  circle A0 centre (0, 0) radius 24.3967
  circle A1 centre (0, 0) radius 26.700373
  point P0 (-9.880865, -22.306221)
  constraints: 2 coincident, 1 centre point, 3 other
extrude "Extrusion2" add sketch "Sketch2" against normal blind 3.81
sketch "Sketch3" plane through (0, 3.81, 0) normal (0, 1, 0) x (1, 0, 0)
  circle A0 centre (0, 0) radius 24.3967
  constraints: 1 centre point, 1 coincident
extrude "Extrusion3" add sketch "Sketch3" against normal blind 2.54
sketch "Sketch4" plane through (0, 3.81, 0) normal (0, 1, 0) x (1, 0, 0)
  circle A0 centre (0, 0) radius 6.35
  dimension "d6" = 12.7
  constraints: 1 centre point, 1 coincident
  measures "d6" diameter of A0
extrude "Extrusion4" cut sketch "Sketch4" against normal blind 2.54
fillet "Fillet1" radius 3.175 8 edges at (29.1925, 1.905, 4.0714) (29.1925, 1.905, -4.0714) (-4.0714, 1.905, -29.1925) (4.0714, 1.905, -29.1925) (-4.0714, 1.905, 29.1925) (-29.1925, 1.905, 4.0714) (4.0714, 1.905, 29.1925) (-29.1925, 1.905, -4.0714)
sketch "Sketch5" plane through (0, 3.81, 0) normal (0, 1, 0) x (1, 0, 0)
  circle A0 centre (0, 33.02) radius 1.778 projected
  circle A1 centre (-33.02, 0) radius 1.778 projected
  circle A2 centre (33.02, 0) radius 1.778 projected
  circle A3 centre (0, -33.02) radius 1.778 projected
  circle A4 centre (0, 33.02) radius 1.905
  circle A5 centre (-33.02, 0) radius 1.905
  circle A6 centre (0, -33.02) radius 1.905
  circle A7 centre (33.02, 0) radius 1.905
  point P0 (0, 0)
  dimension "d10" = 3.81
  dimension "d11" = 3.81
  dimension "d12" = 3.81
  dimension "d13" = 3.81
  constraints: 4 centre point, 4 coincident
  measures "d10" diameter of A4
  measures "d11" diameter of A5
  measures "d12" diameter of A6
  measures "d13" diameter of A7
extrude "Extrusion5" cut sketch "Sketch5" against normal blind 5.08 contours A0 | A1 | A2 | A3 | A4 | A5 | A6 | A7
body "Solid1"
